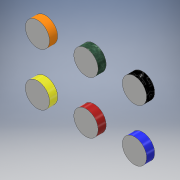
# Autodesk Inventor part: bt
Saved by Autodesk Inventor 2017 (Build 210142000, 142)
## iProperties
Created: 2017-10-10
Part Number: bt
Material: Generic
Document SubType Name: Modeling
Designer: Felipe
Density: 1 g/cm^3
Appearance: Default
Author: Felipe
Autodesk Inventor part; units mm, degrees
ref_plane "YZ Plane" through (0, 0, 0) normal (1, 0, 0) x (0, 1, 0)
ref_plane "XZ Plane" through (0, 0, 0) normal (0, 1, 0) x (-1, 0, 0)
ref_plane "XY Plane" through (0, 0, 0) normal (0, 0, 1) x (1, 0, 0)
sketch "Sketch1" plane through (0, 0, 0) normal (0, 1, 0) x (-1, 0, 0)
  circle A0 centre (0, 0) radius 15
  line L0 (0, 0) -> (47.0979, 0) construction
  circle A1 centre (60, 0) radius 15
  circle A2 centre (120, 0) radius 15
  line L1 (0, 0) -> (0, -192.965) construction
  circle A3 centre (0, -65) radius 15
  line L2 (0, -65) -> (47.0979, -65) construction
  circle A4 centre (60, -65) radius 15
  circle A5 centre (120, -65) radius 15
  dimension "d0" = 30
  dimension "d6" = 60
  dimension "d13" = 65
  constraints: 6 centre point, 6 end point, 2 horizontal, 2 vertical, 1 coincident, 12 other
  measures "d0" diameter of A0
  measures "d6" distance of L0.start A1.centre
  measures "d13" distance of L0.start L2.start
extrude "Extrusion1" add sketch "Sketch1" along normal blind 10
body "Solid1"
